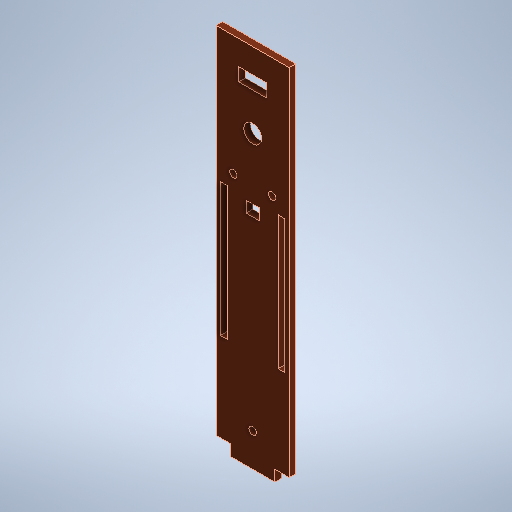
# Autodesk Inventor part: Motor Fixation .1 FV
Saved by Autodesk Inventor 2025.4 (Build 294407000, 407)
## iProperties
Created: 2026-04-11
Part Number: Motor Fixation .1 FV
Material: Generic
Document SubType Name: Sheet Metal
Designer: lenovo
Density: 1 g/cm^3
Sheet Metal Rule: Default_mm
Appearance: Default(1)
Author: lenovo
Autodesk Inventor part; units mm, degrees
ref_plane "YZ Plane" through (0, 0, 0) normal (1, 0, 0) x (0, 1, 0)
ref_plane "XZ Plane" through (0, 0, 0) normal (0, 1, 0) x (-1, 0, 0)
ref_plane "XY Plane" through (0, 0, 0) normal (0, 0, 1) x (1, 0, 0)
sketch "Sketch1" plane through (0, 0, 0) normal (0, 0, 1) x (1, 0, 0)
  line L0 (-16.5, -70) -> (16.5, -70)
  line L1 (16.5, -70) -> (16.5, 70)
  line L2 (16.5, 70) -> (-16.5, 70)
  line L3 (-16.5, 70) -> (-16.5, -70)
  line L4 (-16.5, -70) -> (16.5, 70) construction
  line L5 (16.5, -70) -> (-16.5, 70) construction
  line L6 (0, 70) -> (0, -70)
  line L7 (11.5, 30) -> (14.5, 30)
  line L8 (14.5, 30) -> (14.5, -30)
  line L9 (14.5, -30) -> (11.5, -30)
  line L10 (11.5, -30) -> (11.5, 30)
  line L11 (-11.5, 30) -> (-14.5, 30)
  line L12 (-14.5, -30) -> (-11.5, -30)
  line L13 (-14.5, 30) -> (-14.5, -30)
  line L14 (-11.5, -30) -> (-11.5, 30)
  circle A0 centre (0, -60) radius 1.7
  circle A1 centre (0, 56) radius 10
  line L15 (-10, 56) -> (10, 56)
  line L16 (-6.3196, 63.75) -> (6.3196, 63.75)
  line L17 (-6.3196, 48.25) -> (6.3196, 48.25)
  circle A2 centre (8.75, 36) radius 1.65
  circle A3 centre (-8.75, 36) radius 1.65
  circle A4 centre (0, 56) radius 4
  point P0 (0, 0)
  point P1 (0, 0)
  point P2 (14.5, 0)
  point P3 (16.5, 0)
  point P4 (-14.5, 0)
  point P5 (0, 0)
  point P6 (-6.3196, 48.25)
  point P7 (6.3196, 48.25)
  dimension "d0" = 140
  dimension "d1" = 3
  dimension "d2" = 2
  dimension "d3" = 60
  dimension "d6" = 3.4
  dimension "d7" = 10
  dimension "d9" = 23
  dimension "d13" = 14
  dimension "d14" = 20
  dimension "d15" = 15.5
  dimension "d17" = 3.3
  dimension "d18" = 20
  dimension "d19" = 17.5
  dimension "d22" = 8
  measures "d0" distance of L0.end L2.start
  measures "d1" distance of L7.start L7.end
  measures "d2" distance between parallel lines of L1 L8
  measures "d3" distance of L7.end L9.start
  measures "d6" diameter of A0
  measures "d7" distance from line of L0 A0.centre
  measures "d9" distance between parallel lines of L10 L14
  measures "d13" distance from line of A1.centre L2
  measures "d14" diameter of A1
  measures "d15" diameter of L16 L15
  measures "d17" diameter of A2
  measures "d18" vertical distance of A2.centre A1.centre
  measures "d19" diameter of A2.centre L6
  measures "d22" diameter of A4
extrude "Plate1" add sketch "Sketch1" along normal blind 3 contours L3 L2 L6 A1 A0 L0 | L6 A0 A1 L2 L1 L0 | A1 L16 L6 | L6 L16 A1 | A1 L17 L6 | L6 L17 A1 | L16 A1 L15 A4 L6 | L6 A4 L15 A1 L16 | L17 A1 L15 A4 L6 | L6 A4 L15 A1 L17
sketch "Sketch3" plane through (0, 0, 3) normal (0, 0, 1) x (1, 0, 0)
  line L0 (-16.5, 70) -> (-16.5, -70)
  line L1 (-16.5, 70) -> (16.5, 70)
  line L2 (16.5, 70) -> (16.5, 90)
  line L3 (16.5, 90) -> (-16.5, 90)
  line L4 (-16.5, 90) -> (-16.5, 70)
  line L5 (-16.5, 0) -> (16.5, 0)
  line L6 (16.5, -70) -> (16.5, 70)
  point P0 (0, 0)
  dimension "d23" = 20
  measures "d23" distance of L1.end L2.end
sheet face with bend "Face2" sketch "Sketch3" thickness 3 toward (0, 0, -1) bend radius 3 contours L4 L3 L2 L1
bend "Bend1"
sketch "Sketch4" plane through (0, 0, 3) normal (0, 0, 1) x (1, 0, 0)
  line L0 (-10, -70) -> (10, -70)
  line L1 (10, -70) -> (10, -75)
  line L2 (10, -75) -> (-10, -75)
  line L3 (-10, -75) -> (-10, -70)
  line L4 (16.5, -70) -> (-16.5, -70)
  point P0 (0, 0)
  point P1 (0, -70)
  point P2 (0, -70)
  point P3 (0, -70)
  dimension "d29" = 20
  dimension "d30" = 5
  measures "d29" distance of L1.end L2.end
  measures "d30" distance of L0.end L1.end
sheet face with bend "Face3" sketch "Sketch4" thickness 3 toward (0, 0, -1) bend radius 3
bend "Bend2"
sketch "Sketch5" plane through (0, 0, 3) normal (0, 0, 1) x (1, 0, 0)
  line L0 (-3, 23.5) -> (3, 23.5)
  line L1 (3, 23.5) -> (3, 28.5)
  line L2 (3, 28.5) -> (-3, 28.5)
  line L3 (-3, 28.5) -> (-3, 23.5)
  line L4 (-3, 23.5) -> (3, 28.5) construction
  line L5 (3, 23.5) -> (-3, 28.5) construction
  circle A0 centre (0, 56) radius 4 projected
  point P0 (0, 0)
  point P1 (0, 26)
  dimension "d36" = 6
  dimension "d37" = 5
  dimension "d38" = 30
  constraints: 12 end point, 2 midpoint, 2 parallel, 1 horizontal, 1 perpendicular, 1 vertical alignment
  measures "d36" distance of L1.end L2.end
  measures "d37" distance of L0.end L1.end
  measures "d38" distance of A0.centre point (0, 26)
extrude "Cut1" cut sketch "Sketch5" against normal blind 3 contours L3 L2 L1 L0
sketch "Sketch6" plane through (0, 0, 3) normal (0, 0, 1) x (1, 0, 0)
  line L0 (-6.325, 78.95) -> (6.325, 78.95)
  line L1 (6.325, 78.95) -> (6.325, 73.05)
  line L2 (6.325, 73.05) -> (-6.325, 73.05)
  line L3 (-6.325, 73.05) -> (-6.325, 78.95)
  line L4 (-6.325, 78.95) -> (6.325, 73.05) construction
  line L5 (6.325, 78.95) -> (-6.325, 73.05) construction
  circle A0 centre (0, 56) radius 4 projected
  point P0 (0, 0)
  point P1 (0, 76)
  dimension "d41" = 12.65
  dimension "d42" = 5.9
  dimension "d43" = 20
  constraints: 12 end point, 2 midpoint, 2 parallel, 1 horizontal, 1 perpendicular, 1 vertical alignment
  measures "d41" distance of L1.end L2.end
  measures "d42" distance between parallel lines of L0 L2
  measures "d43" distance of point (0, 76) A0.centre
extrude "Cut2" cut sketch "Sketch6" against normal blind 3 contours L0 L1 L2 L3
equation "\"d39\" = Thickness"
equation "\"d44\" = Thickness"
equation "\"d16\" = Thickness"
equation "\"d24\" = BendRadius"
equation "\"d25\" = BendReliefWidth"
equation "\"d27\" = MinimumRemnant"
equation "\"d26\" = BendReliefDepth"
equation "\"d28\" = TransitionRadius"
equation "\"d31\" = BendRadius"
equation "\"d32\" = BendReliefWidth"
equation "\"d34\" = MinimumRemnant"
equation "\"d33\" = BendReliefDepth"
equation "\"d35\" = TransitionRadius"
equation "\"BendRadius\" = Thickness"
equation "\"BendReliefWidth\" = Thickness"
equation "\"BendReliefDepth\" = 0.5 * Thickness"
equation "\"CornerReliefSize\" = 4 * Thickness"
equation "\"MinimumRemnant\" = 2 * Thickness"
equation "\"TransitionRadius\" = BendRadius"
equation "\"JacobiRadiusSize\" = BendRadius"
equation "\"GapSize\" = Thickness"
equation "\"Thickness\" = 3"
body "Solid1"
